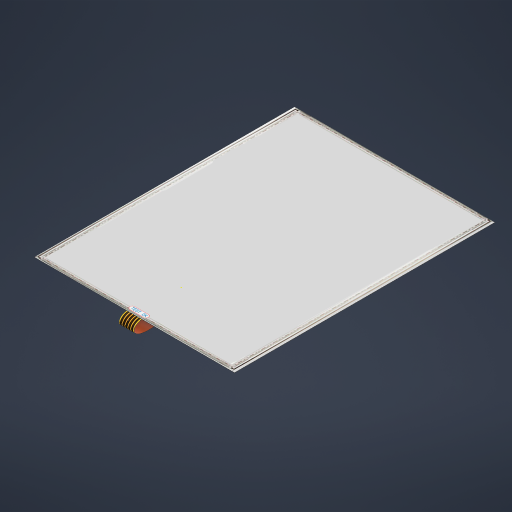
# Autodesk Inventor part: 12inch Touchscreen
Saved by Autodesk Inventor 2023 (Build 270158000, 158)
## iProperties
Created: 2023-02-24
Part Number: 12inch Touchscreen
Material: Generic
Document SubType Name: Modeling
Designer: roota
Density: 1 g/cm^3
Appearance: Default
Author: roota
Autodesk Inventor part; units mm, degrees
ref_plane "YZ Plane" through (0, 0, 0) normal (1, 0, 0) x (0, 1, 0)
ref_plane "XZ Plane" through (0, 0, 0) normal (0, 1, 0) x (-1, 0, 0)
ref_plane "XY Plane" through (0, 0, 0) normal (0, 0, 1) x (1, 0, 0)
sketch "Sketch1" plane through (0, 0, 0) normal (0, 1, 0) x (-1, 0, 0)
  line L0 (100, 130) -> (-100, 130)
  line L1 (-100, 130) -> (-100, -130)
  line L2 (-100, -130) -> (100, -130)
  line L3 (100, -130) -> (100, 130)
  line L4 (100, 130) -> (-100, -130) construction
  line L5 (-100, 130) -> (100, -130) construction
  point P0 (0, 0)
  dimension "d0" = 200
  dimension "d1" = 260
  constraints: 12 end point, 2 midpoint, 2 parallel, 1 horizontal, 1 perpendicular
  measures "d0" distance of L2.end L1.end
  measures "d1" distance of L1.end L0.end
extrude "Extrusion1" add sketch "Sketch1" along normal blind 0.188
sketch "Sketch2" plane through (0, 0, 0) normal (1, 0, 0) x (0, 1, 0)
  line L0 (0.188, 130) -> (0.188, -130) projected
  line L1 (0, 90.3171) -> (0, 130) construction
  spline S0 degree 4 poles (0, 130) (0, 134.3554) (-9.058, 147.1635) (-19.4629, 125.986) (-6.9491, 96.3654) (-6.9491, 83.2036) knots 0 0 0 0 0 0.420838 1 1 1 1 1
  line L2 (0, 130) -> (0, 216.7) construction
  line L3 (-6.9491, 83.2036) -> (-6.9491, 68.2036) construction
  point P0 (0, 0)
  point P1 (-4.7515, 137.602)
  point P2 (-10.9897, 132.9238)
  dimension "d4" = 86.7
  dimension "d10" = 15
  constraints: 6 end point, 5 vertical, 1 coincident, 4 other
  measures "d4" distance of L1.end L2.end
  measures "d10" distance of L3.start L3.end
sketch "Sketch3" plane through (0, 0, 0) normal (1, 0, 0) x (0, 1, 0)
  spline S0 degree 4 poles (0, 130) (0, 134.3554) (-9.058, 147.1635) (-19.4629, 125.986) (-6.9491, 96.3654) (-6.9491, 83.2036) knots 0 0 0 0 0 0.420838 1 1 1 1 1 projected
  line L0 (0, 130) -> (0, -130) projected
  line L1 (0, 130) -> (0.1, 130)
  line L2 (0, 130) -> (0.188, 130) projected
  line L3 (-6.9491, 83.2036) -> (-7.0491, 83.2036)
  spline S1 degree 5 poles (0.1, 130) (0.0999, 130.7955) (-0.017, 131.59) (-0.2179, 132.3644) (-0.7518, 133.8269) (-1.5556, 135.1608) (-2.0069, 135.7697) (-2.9646, 136.7997) (-4.1564, 137.5331) (-4.7543, 137.7888) (-6.0479, 138.0417) (-7.3301, 137.7194) (-7.9234, 137.4064) (-9.1636, 136.4634) (-10.0681, 135.1789) (-10.4986, 134.3925) (-11.3561, 132.458) (-11.892, 130.4092) (-12.125, 129.2139) (-12.5034, 126.5067) (-12.614, 123.774) (-12.6116, 122.2573) (-12.4936, 118.99) (-12.1719, 115.7362) (-11.9542, 113.9967) (-11.4264, 110.3923) (-10.7785, 106.8075) (-10.4202, 104.9519) (-9.6766, 101.2403) (-8.9234, 97.5307) (-8.5548, 95.6714) (-7.8843, 92.0804) (-7.367, 88.4639) (-7.1705, 86.7171) (-7.0491, 84.9606) (-7.0491, 83.2036) knots 0 0 0 0 0 0 0.057808 0.057808 0.057808 0.112654 0.112654 0.112654 0.158866 0.158866 0.158866 0.206246 0.206246 0.206246 0.271253 0.271253 0.271253 0.359601 0.359601 0.359601 0.469759 0.469759 0.469759 0.597143 0.597143 0.597143 0.734514 0.734514 0.734514 0.872293 0.872293 0.872293 1 1 1 1 1 1
  point P0 (0, 0)
  dimension "d5" = 0.1
  constraints: 4 end point, 1 collinear, 1 horizontal, 3 other
extrude "Extrusion2" add sketch "Sketch3" along normal mid plane 15
sketch "Sketch4" plane through (-7.5, -37.8125, 83.2036) normal (0, 0, -1) x (1, 0, 0)
  line L0 (0, -30.8634) -> (0, -30.7634) projected
  line L1 (0, -30.7634) -> (15, -30.7634) projected
  line L2 (0, -30.8634) -> (15, -30.8634)
  line L3 (15, -30.8634) -> (15, -30.7634)
  line L4 (15, -30.7634) -> (0, -30.7634)
  line L5 (0, -30.7634) -> (0, -30.8634)
  point P0 (7.5, -37.8125)
  constraints: 8 end point, 2 parallel, 1 horizontal, 1 perpendicular
extrude "Extrusion3" add sketch "Sketch4" along normal blind 20
sketch "Sketch5" plane through (0, 0.188, 0) normal (0, 1, 0) x (1, 0, 0)
  line L0 (7.5, -44.1487) -> (7.5, -140.6515) construction
  line L1 (7.5, -140.6515) -> (-7.5, -140.6515) construction
  line L2 (-7.5, -140.6515) -> (-7.5, -44.1487) construction
  line L3 (-7.5, -44.1487) -> (7.5, -44.1487) construction
  point P0 (0, 0)
  point P1 (7.5, -130)
  point P2 (-7.5, -130)
  constraints: 2 vertical alignment, 2 other
decal "Decal1"
sketch "Sketch6" plane through (-7.5, -7.0491, 83.2036) normal (0, -1, 0) x (1, 0, 0)
  line L0 (0.0146, -20.011) -> (0, 0) construction
  line L1 (0, 0) -> (14.9854, 0.011) construction
  line L2 (14.9854, 0.011) -> (15, -20) construction
  line L3 (15, -20) -> (0.0146, -20.011) construction
  point P0 (7.5, -83.2036)
  point P1 (15, -20)
  constraints: 2 coincident, 2 other
decal "Decal2"
sketch "Sketch7" plane through (7.5, -6.9491, 83.2036) normal (0, 1, 0) x (-1, 0, 0)
  line L0 (0.0146, -20.011) -> (0, 0) construction
  line L1 (0, 0) -> (14.9854, 0.011) construction
  line L2 (14.9854, 0.011) -> (15, -20) construction
  line L3 (15, -20) -> (0.0146, -20.011) construction
  point P0 (7.5, -83.2036)
  point P1 (15, -20)
  constraints: 2 coincident, 2 other
decal "Decal3"
sketch "Sketch8" plane through (0, 0, 0) normal (0, -1, 0) x (1, 0, 0)
  line L0 (7.5, 207.6879) -> (7.5, 130) construction
  line L1 (7.5, 130) -> (-7.5, 130) construction
  line L2 (-7.5, 130) -> (-7.5, 207.6879) construction
  line L3 (-7.5, 207.6879) -> (7.5, 207.6879) construction
  point P0 (0, 0)
  constraints: 2 coincident, 2 other
decal "Decal4"
sketch "Sketch10" plane through (0, 0.188, 0) normal (0, 1, 0) x (1, 0, 0)
  line L0 (98.0274, 130) -> (98.0274, -130) construction
  line L1 (98.0274, -130) -> (-100, -130) construction
  line L2 (-100, -130) -> (-100, 130) construction
  line L3 (-100, 130) -> (98.0274, 130) construction
  point P0 (0, 0)
  constraints: 2 coincident, 2 other
decal "Decal6"
sketch "Sketch11" plane through (0, 0, 0) normal (0, -1, 0) x (1, 0, 0)
  line L0 (-98.7516, -130.9508) -> (-100, 130) construction
  line L1 (-100, 130) -> (98.7516, 130.9508) construction
  line L2 (98.7516, 130.9508) -> (100, -130) construction
  line L3 (100, -130) -> (-98.7516, -130.9508) construction
  point P0 (0, 0)
  constraints: 2 coincident, 2 other
decal "Decal7"
sketch "Sketch9" plane through (0, 0.188, 0) normal (0, 1, 0) x (1, 0, 0)
  line L0 (-9.9844, -128.5553) -> (-9.9844, -122.1467) construction
  line L1 (-9.9844, -122.1467) -> (9.7409, -122.1467) construction
  line L2 (9.7409, -122.1467) -> (9.7409, -128.5553) construction
  line L3 (9.7409, -128.5553) -> (-9.9844, -128.5553) construction
  point P0 (0, 0)
  constraints: 2 other
decal "Decal5"
sketch "Sketch12" plane through (0, 0, 0) normal (1, 0, 0) x (0, 1, 0)
  line L0 (-36.5283, 83.3447) -> (-6.2422, 162.4124)
  line L1 (-36.5283, 83.3447) -> (-63.1781, 93.5527)
  point P0 (0, 0)
  constraints: 4 end point
ref_plane "Work Plane1" through (0, -36.5283, 83.3447) normal (0, -0.9338373, 0.3576979) x (1, 0, 0)
sketch "Sketch13" plane through (0, -36.5283, 83.3447) normal (0, -0.9338373, 0.3576979) x (1, 0, 0)
  line L0 (7.5, 88.1007) -> (7.5, 10.4128) construction
  line L1 (7.5, 10.4128) -> (-7.5, 10.4128) construction
  line L2 (-7.5, 10.4128) -> (-7.5, 88.1007) construction
  line L3 (-7.5, 88.1007) -> (7.5, 88.1007) construction
  point P0 (0, -64.7643)
  constraints: 2 coincident, 2 other
decal "Decal8"
body "Solid1"
